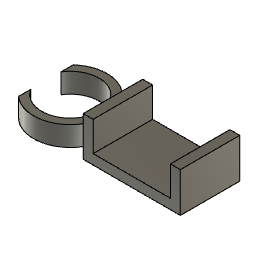
doorHolder (Autodesk Fusion 360 design; units mm, degrees)
Autodesk Fusion 360 part; units mm, degrees
sketch "doorStop" plane through (0, 0, 0) normal (0, 0, 1) x (1, 0, 0)
  circle A0 centre (0, 0) radius 18.5
  circle A1 centre (0, 0) radius 14.5
  line L0 (0, 0) -> (-12.325, 0) construction
  line L1 (-12.325, 0) -> (-14.5, 0)
  line L2 (-14.5, 0) -> (-14.5, 16.5)
  line L3 (-14.5, 16.5) -> (-12.325, 16.5)
  line L4 (-12.325, 16.5) -> (-12.325, 0)
  line L5 (-12.325, 0) -> (-14.5, 0)
  line L6 (-14.5, 0) -> (-14.5, -16.5)
  line L7 (-14.5, -16.5) -> (-12.325, -16.5)
  line L8 (-12.325, -16.5) -> (-12.325, 0)
  dimension "d4" = 37
  dimension "d5" = 29
  dimension "d6" = 12.325
  dimension "d7" = 2.175
  dimension "d8" = 16.5
  dimension "d9" = 2.175
  dimension "d10" = 16.5
  constraint coincident A0.centre A1.centre
  constraint horizontal L0
  constraint horizontal L1
  constraint vertical L2
  constraint horizontal L3
  constraint vertical L4
  constraint horizontal L5
  constraint vertical L6
  constraint horizontal L7
  constraint vertical L8
  measures "d4" diameter of A0
  measures "d5" diameter of A1
  measures "d6" distance of A0.centre L0.end
  measures "d7" distance of L0.end L1.end
  measures "d8" distance of L0.end L3.end
  measures "d9" distance of L0.end L1.end
  measures "d10" distance of L0.end L7.end
extrude "Extrude1" add sketch "doorStop" along normal blind 10 contours A0 A1 L4 L8 makes body 1
ref_plane "WorkPlane3" through (18.5, 0, 8.3668) normal (1, 0, 0) x (0, -1, 0)
sketch "link" plane through (18.5, 0, 7.5753) normal (1, 0, 0) x (0, 1, 0)
  line L0 (-13.7965, -7.5753) -> (-7.6383, -7.5753)
  line L1 (-7.6383, 2.4247) -> (-13.7965, 2.4247)
  line L2 (-7.6383, -7.5753) -> (7.6383, -7.5753)
  line L3 (7.6383, 2.4247) -> (-7.6383, 2.4247)
  line L4 (13.7965, -7.5753) -> (7.6383, -7.5753)
  line L5 (13.7965, 2.4247) -> (7.6383, 2.4247)
  line L6 (-13.7965, -7.5753) -> (-18.5, -7.5753)
  line L7 (18.5, -7.5753) -> (13.7965, -7.5753)
  line L8 (-13.7965, 2.4247) -> (-18.5, 2.4247)
  line L9 (18.5, 2.4247) -> (13.7965, 2.4247)
  line L10 (18.5, -7.5753) -> (18.5, 2.4247)
  line L11 (-18.5, -7.5753) -> (-18.5, 2.4247)
  line L12 (-18.5, -7.5753) -> (18.5, -7.5753) construction
  line L13 (-18.5, -7.5753) -> (18.5, -7.5753) construction
  line L14 (0, -7.5753) -> (-5, -7.5753) construction
  line L15 (-5, -7.5753) -> (5, -7.5753)
  line L16 (5, -7.5753) -> (5, 2.4247)
  line L17 (5, 2.4247) -> (-5, 2.4247)
  line L18 (-5, 2.4247) -> (-5, -7.5753)
  point P0 (0, -7.5753)
  dimension "d20" = 5
  dimension "d21" = 10
  dimension "d22" = 10
  constraint coincident L6.end L11.start
  constraint coincident L7.start L10.start
  constraint coincident L2 P0
  constraint midpoint L12 P0
  constraint coincident P0 L14.start
  constraint parallel L12 L14
  constraint horizontal L15
  constraint vertical L16
  constraint horizontal L17
  constraint vertical L18
  measures "d20" distance of P0 L14.end
  measures "d21" distance of L14.end L15.end
  measures "d22" distance of L14.end L17.end
extrude "Extrude2" add sketch "link" along normal blind 3 separate body contours L2 L3 L15 L16 L17 L18 makes body 2
extrude "Extrude3" add 1 faces at (18.5, -1.6667, 6.6667) along direction (-1, 0, 0) blind 1 on bodies 2 bodies 2 1
ref_plane "WorkPlane4" through (21.5, 0, 5) normal (1, 0, 0) x (0, 0, -1)
sketch "doorHolder1" plane through (21.5, 0, 2.5) normal (1, 0, 0) x (0, 1, 0)
  line L0 (-5, 7.5) -> (-5, -2.5)
  line L1 (-5, -2.5) -> (5, -2.5)
  line L2 (5, -2.5) -> (5, 7.5)
  line L3 (5, 7.5) -> (-5, 7.5)
  line L4 (-5, -2.5) -> (5, -2.5) construction
  line L5 (0, -2.5) -> (-15, -2.5) construction
  line L6 (-15, -2.5) -> (15, -2.5)
  line L7 (15, -2.5) -> (15, 17.5)
  line L8 (15, 17.5) -> (-15, 17.5)
  line L9 (-15, 17.5) -> (-15, -2.5)
  point P0 (0, -2.5)
  dimension "d31" = 15
  dimension "d32" = 30
  dimension "d33" = 20
  constraint coincident L0.end L1.start
  constraint coincident L1.end L2.start
  constraint coincident L1 P0
  constraint midpoint L4 P0
  constraint coincident P0 L5.start
  constraint perpendicular L0 L5
  constraint horizontal L6
  constraint vertical L7
  constraint horizontal L8
  constraint vertical L9
  measures "d31" distance of P0 L5.end
  measures "d32" distance of L5.end L6.end
  measures "d33" distance of L5.end L8.end
extrude "Extrude4" add sketch "doorHolder1" along normal blind 5 bodies 2
ref_plane "WorkPlane5" through (26.5, 0, 10) normal (1, 0, 0) x (0, 0, -1)
sketch "doorHolderBottom" plane through (26.5, 0, 10) normal (1, 0, 0) x (0, 1, 0)
  line L0 (-15, 10) -> (-15, -10)
  line L1 (-15, -10) -> (15, -10)
  line L2 (15, -10) -> (15, 10)
  line L3 (15, 10) -> (-15, 10)
  line L4 (-15, -10) -> (15, -10)
  line L5 (15, -10) -> (15, -5)
  line L6 (15, -5) -> (-15, -5)
  line L7 (-15, -5) -> (-15, -10)
  dimension "d37" = 30
  dimension "d38" = 5
  constraint horizontal L4
  constraint vertical L5
  constraint horizontal L6
  constraint vertical L7
  constraint coincident L0.end L1.start
  measures "d37" distance of L0.end L1.end
  measures "d38" distance of L0.end L6.end
extrude "Extrude5" add sketch "doorHolderBottom" along normal blind 39 contours L0 L1 L2 L4 L5 L6 L7 bodies 2
ref_plane "WorkPlane6" through (65.5, 0, 2.5) normal (1, 0, 0) x (0, 0, -1)
sketch "doorHolder2" plane through (65.5, 0, 2.5) normal (1, 0, 0) x (0, 1, 0)
  line L0 (0, -2.5) -> (-15, -2.5) construction
  line L1 (-15, -2.5) -> (15, -2.5)
  line L2 (15, 17.5) -> (-15, 17.5)
  line L3 (15, -2.5) -> (15, 17.5)
  line L4 (-2.5, 2.5) -> (-2.5, -2.5)
  line L5 (-15, 17.5) -> (-15, -2.5)
  line L6 (2.5, 2.5) -> (-2.5, 2.5)
  line L7 (-2.5, -2.5) -> (2.5, -2.5) construction
  line L8 (2.5, -2.5) -> (2.5, 2.5)
  line L9 (-2.5, -2.5) -> (2.5, -2.5)
  point P0 (0, -2.5)
  dimension "d43" = 15
  dimension "d44" = 30
  dimension "d45" = 20
  constraint coincident L4.end L7.start
  constraint coincident L7.end L8.start
  constraint coincident P0 L9
  constraint midpoint P0 L7
  constraint coincident P0 L0.start
  constraint perpendicular L0 L4
  constraint horizontal L1
  constraint vertical L3
  constraint horizontal L2
  constraint vertical L5
  measures "d43" distance of L0.end P0
  measures "d44" distance of L0.end L1.end
  measures "d45" distance of L0.end L2.end
extrude "Extrude6" add sketch "doorHolder2" along normal blind 5 bodies 2
equation "doorStopDiameter = 29 mm"
equation "doorStopHolderThickness = 4 mm"
equation "d4 = doorStopDiameter + ( 2 * doorStopHolderThickness )"
equation "d5 = doorStopDiameter"
equation "d6 = ( doorStopDiameter / 2 ) * ( doorStopHolderClosurePercent )"
equation "d7 = ( doorStopDiameter / 2 ) * ( 1 - doorStopHolderClosurePercent )"
equation "d8 = ( doorStopDiameter + doorStopHolderThickness ) / 2"
equation "d9 = ( doorStopDiameter / 2 ) * ( 1 - doorStopHolderClosurePercent )"
equation "d10 = ( doorStopDiameter + doorStopHolderThickness ) / 2"
equation "d11 = doorStopHeight"
equation "doorStopHeight = 10 mm"
equation "linkLength = 3 mm"
equation "linkThickness = 10 mm"
equation "d20 = linkThickness / 2"
equation "d21 = linkThickness"
equation "d22 = doorStopHeight"
equation "d23 = linkLength"
equation "doorHolderHeight = 15 mm"
equation "doorHolderWidth = 30 mm"
equation "doorHolderThickness = 5 mm"
equation "d31 = doorHolderWidth / 2"
equation "d32 = doorHolderWidth"
equation "d33 = doorHolderHeight + doorHolderThickness"
equation "d34 = doorHolderThickness"
equation "d37 = doorHolderWidth"
equation "d38 = doorHolderThickness"
equation "d39 = doorThickness"
equation "doorThickness = 39 mm"
equation "d43 = doorHolderWidth / 2"
equation "d44 = doorHolderWidth"
equation "d45 = doorHolderHeight + doorHolderThickness"
equation "d46 = doorHolderThickness"
equation "doorStopHolderClosurePercent = 0.85"
